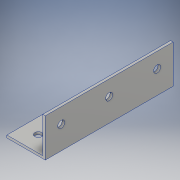
# Autodesk Inventor part: Column Mount
Saved by Autodesk Inventor 2019.4 (Build 234330000, 330)
## iProperties
Created: 2020-01-24
Part Number: Column Mount
Material: Aluminum 6061
Document SubType Name: Modeling
Designer: admin
Density: 2.7 g/cm^3
Appearance: Aluminum - Flat
Author: admin
Autodesk Inventor part; units mm, degrees
ref_plane "YZ Plane" through (0, 0, 0) normal (1, 0, 0) x (0, 1, 0)
ref_plane "XZ Plane" through (0, 0, 0) normal (0, 1, 0) x (-1, 0, 0)
sketch "Sketch1" plane through (0, 0, 0) normal (0, 0, 1) x (1, 0, 0)
  line L0 (0, 0) -> (0, 30)
  line L1 (0, 30) -> (-2, 30)
  line L2 (-2, 30) -> (-2, 2)
  line L3 (-2, 2) -> (-30, 2)
  line L4 (-30, 2) -> (-30, 0)
  line L5 (-30, 0) -> (0, 0)
  dimension "d0" = 2
  dimension "d1" = 2
  dimension "d2" = 30
  dimension "d3" = 30
  constraints: 12 end point, 5 perpendicular, 1 vertical
  measures "d0" distance between parallel lines of L5 L3
  measures "d1" distance between parallel lines of L0 L2
  measures "d2" distance of L4.end L0.start
  measures "d3" distance of L0.start L0.end
extrude "Extrusion1" add sketch "Sketch1" along normal blind 100
sketch "Sketch2" plane through (-30, 2, 0) normal (0, 1, 0) x (1, 0, 0)
  circle A0 centre (12, -12.5) radius 2.75
  circle A1 centre (12, -87.5) radius 2.75
  circle A2 centre (12, -50) radius 2.75
  line L0 (12, -87.5) -> (12, -12.5) construction
  line L1 (0, 0) -> (0, -100) projected
  line L2 (12, -50) -> (0, -50) construction
  point P0 (30, 0)
  dimension "d6" = 5.5
  dimension "d7" = 5.5
  dimension "d8" = 5.5
  dimension "d9" = 12
  dimension "d10" = 75
  constraints: 4 end point, 3 centre point, 2 midpoint, 1 coincident, 1 perpendicular, 1 vertical
  measures "d6" diameter of A0
  measures "d7" diameter of A1
  measures "d8" diameter of A2
  measures "d9" distance between parallel lines of L1 L0
  measures "d10" distance of L0.start L0.end
extrude "Extrusion2" cut sketch "Sketch2" against normal through all
ref_plane "Work Plane1" through (-2, 2, 0) normal (0.7071, 0.7071, 0) x (0, 0, 1)
mirror "Mirror1" about plane through (-2, 2, 0) normal (0.7071, 0.7071, 0) of "Extrusion2"
body "Solid1"
